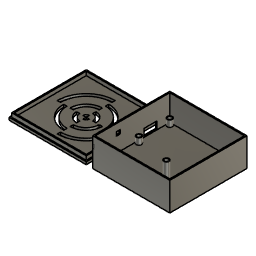
Fujitsu case new v2 (Autodesk Fusion 360 design; units mm, degrees)
Autodesk Fusion 360 part; units mm, degrees
note: some values were not read from the file. Set by a fixed rule: which sketch regions a step uses.
sketch "Sketch1" plane through (0, 0, 0) normal (0, 0, 1) x (1, 0, 0)
  line L0 (30, -30) -> (-30, -30)
  line L1 (-30, -30) -> (-30, 30)
  line L2 (-30, 30) -> (30, 30)
  line L3 (30, 30) -> (30, -30)
  line L4 (30, -30) -> (-30, 30) construction
  line L5 (-30, -30) -> (30, 30) construction
  dimension "d1" = 60
  dimension "d2" = 60
  constraint horizontal L0
  constraint perpendicular L0 L1
  constraint parallel L0 L2
  constraint parallel L1 L3
  constraint coincident L4 origin
  constraint coincident L5 origin
  measures "d1" distance of L1.end L2.end
  measures "d2" distance of L0.end L1.end
extrude "Extrude1" add sketch "Sketch1" along normal blind 2 makes body 1
sketch "Sketch2" plane through (0, 0, 2) normal (0, 0, 1) x (-1, 0, 0)
  line L0 (-30, -30) -> (30, -30)
  line L1 (30, -30) -> (30, 30)
  line L2 (30, 30) -> (-30, 30)
  line L3 (-30, 30) -> (-30, -30)
  line L4 (30, -30) -> (-30, -30)
  line L5 (-30, -30) -> (-30, 30)
  line L6 (-30, 30) -> (30, 30)
  line L7 (30, 30) -> (30, -30)
  line L8 (29, -29) -> (-29, -29)
  line L9 (-29, -29) -> (-29, 29)
  line L10 (-29, 29) -> (29, 29)
  line L11 (29, 29) -> (29, -29)
  constraint horizontal L4
  constraint vertical L5
  constraint horizontal L6
  constraint vertical L7
  constraint coincident L2.end L3.start
  constraint coincident L0.end L1.start
  constraint horizontal L8
  constraint vertical L9
  constraint horizontal L10
  constraint vertical L11
extrude "Extrude2" add sketch "Sketch2" along normal blind 20 bodies 1
sketch "Sketch3" plane through (0, 0, 2) normal (0, 0, 1) x (-1, 0, 0)
  line L0 (-29, 29) -> (-29, -29)
  line L1 (-29, -29) -> (29, -29)
  line L2 (29, -29) -> (29, 29)
  line L3 (29, 29) -> (-29, 29)
  circle A0 centre (27, -27) radius 2
  circle A1 centre (27, -27) radius 1.5
  line L4 (27, -27) -> (27, -3)
  circle A2 centre (27, -3) radius 1.5
  circle A3 centre (27, -3) radius 2
  line L5 (27, -27) -> (-19, -27)
  circle A4 centre (-19, -27) radius 1.5
  circle A5 centre (-19, -27) radius 2
  line L6 (27, -3) -> (-19, -3)
  circle A6 centre (-19, -3) radius 1.5
  circle A7 centre (-19, -3) radius 2
  dimension "d7" = 4
  dimension "d8" = 3
  dimension "d9" = 24
  dimension "d10" = 3
  dimension "d11" = 4
  dimension "d12" = 46
  dimension "d13" = 3
  dimension "d14" = 4
  dimension "d15" = 46
  dimension "d16" = 3
  dimension "d17" = 4
  constraint concentric A0 A1
  constraint coincident A0.centre A1.centre
  constraint parallel L2 L4
  constraint coincident L4.end A2.centre
  constraint concentric A2 A3
  constraint perpendicular L4 L5
  constraint coincident L5.end A4.centre
  constraint concentric A4 A5
  constraint perpendicular L4 L6
  constraint coincident L6.end A6.centre
  constraint concentric A6 A7
  measures "d7" diameter of A0
  measures "d8" diameter of A1
  measures "d9" distance of A0.centre L4.end
  measures "d10" diameter of A2
  measures "d11" diameter of A3
  measures "d12" distance of A0.centre L5.end
  measures "d13" diameter of A4
  measures "d14" diameter of A5
  measures "d15" distance of L4.end L6.end
  measures "d16" diameter of A6
  measures "d17" diameter of A7
extrude "Extrude3" add sketch "Sketch3" along normal blind 5 separate body contours A5 | L4 A2 A3 L6 | A0 A1 L4 L5 | L4 A2 A3 L6 | A0 A1 L4 L5 | A7 makes body 2 at (-28.9901, 3.1991, 3.6667) makes body 3 at (-28.9901, 27.1991, 3.6667) makes body 4 at (17.0025, 3.0997, 5.3333) makes body 5 at (17.0099, 27.1991, 3.6667)
sketch "Sketch4" plane through (-30, 0, 0) normal (-1, 0, 0) x (0, -1, 0)
  line L0 (-30, 0) -> (30, 0)
  line L1 (30, 0) -> (30, 22)
  line L2 (30, 22) -> (-30, 22)
  line L3 (-30, 22) -> (-30, 0)
  line L4 (-30, 0) -> (-14, 0)
  line L5 (-14, 0) -> (-14, 7)
  line L6 (-14, 7) -> (-14, 7.5)
  line L7 (-14, 7.5) -> (-19, 7.5)
  line L8 (-19, 7.5) -> (-9, 7.5)
  line L9 (-9, 7.5) -> (-9, 2.5)
  line L10 (-9, 2.5) -> (-19, 2.5)
  line L11 (-19, 2.5) -> (-19, 7.5)
  dimension "d20" = 16
  dimension "d21" = 7
  dimension "d22" = 0.5
  dimension "d23" = 5
  dimension "d24" = 10
  dimension "d25" = 5
  constraint coincident L0.start L3.end
  constraint perpendicular L3 L4
  constraint perpendicular L4 L5
  constraint parallel L5 L6
  constraint perpendicular L6 L7
  constraint horizontal L8
  constraint vertical L9
  constraint horizontal L10
  constraint vertical L11
  measures "d20" distance of L0.start L4.end
  measures "d21" distance of L4.end L5.end
  measures "d22" distance of L5.end L6.end
  measures "d23" distance of L6.end L7.end
  measures "d24" distance of L7.end L8.end
  measures "d25" distance of L7.end L10.end
extrude "Extrude4" cut sketch "Sketch4" against normal blind 1 contours L5 L6 L7 L8 L10 L11 | L5 L6 L8 L9 L10 bodies 1
extrude "Extrude5" cut 1 faces at (-29.6667, 15.6667, 7.5) along direction (0, 0, 1) blind 0.5 on bodies 1 bodies 1
sketch "Sketch5" plane through (0, 0, 2) normal (0, 0, 1) x (-1, 0, 0)
  line L0 (-29, 29) -> (-29, -29)
  line L1 (-29, -29) -> (29, -29)
  line L2 (29, -29) -> (29, 29)
  line L3 (29, 29) -> (-29, 29)
  line L4 (22, 29) -> (29, 29)
  line L5 (22, 29) -> (22, 27)
  circle A0 centre (22, 27) radius 2
  circle A1 centre (22, 27) radius 1.5
  line L6 (29, 29) -> (29, 11)
  line L7 (29, 11) -> (-7.9977, 10.5843)
  circle A2 centre (-7.9977, 10.5843) radius 1.5
  circle A3 centre (-7.9977, 10.5843) radius 2
  dimension "d31" = 7
  dimension "d32" = 2
  dimension "d33" = 4
  dimension "d34" = 3
  dimension "d35" = 18
  dimension "d37" = 37
  dimension "d38" = 3
  dimension "d39" = 4
  constraint coincident L2.end L3.start
  constraint perpendicular L2 L4
  constraint perpendicular L4 L5
  constraint coincident L5.end A0.centre
  constraint concentric A0 A1
  constraint perpendicular L4 L6
  constraint coincident L7.end A2.centre
  constraint concentric A2 A3
  measures "d31" distance of L4.start L2.end
  measures "d32" distance of L4.start L5.end
  measures "d33" diameter of A0
  measures "d34" diameter of A1
  measures "d35" distance of L2.end L6.end
  measures "d37" distance of L6.end L7.end
  measures "d38" diameter of A2
  measures "d39" diameter of A3
extrude "Extrude6" add sketch "Sketch5" along normal blind 13 separate body contours A0 | A3 makes body 6 at (-23.9975, -26.9003, 6.3333) makes body 7 at (6.0076, -10.7834, 10.6667)
sketch "Sketch6" plane through (0, 0, 2) normal (0, 0, 1) x (-1, 0, 0)
  line L0 (-29, 29) -> (-29, -29)
  line L1 (-29, -29) -> (29, -29)
  line L2 (29, -29) -> (29, 29)
  line L3 (29, 29) -> (-29, 29)
  line L4 (29, 29) -> (2, 29)
  line L5 (2, 29) -> (2, 26)
  circle A0 centre (2, 26) radius 1.5
  dimension "d42" = 27
  dimension "d43" = 3
  dimension "d44" = 3
  constraint coincident L2.end L3.start
  constraint perpendicular L2 L4
  constraint perpendicular L3 L5
  constraint coincident L5.end A0.centre
  measures "d42" distance of L2.end L4.end
  measures "d43" distance of L4.end L5.end
  measures "d44" diameter of A0
extrude "Extrude7" cut sketch "Sketch6" against normal blind 5 contours A0 bodies 1
sketch "Sketch7" plane through (-30, 0, 0) normal (-1, 0, 0) x (0, -1, 0)
  line L0 (-9, 8) -> (-9, 2.5)
  line L1 (-9, 2.5) -> (-19, 2.5)
  line L2 (-19, 2.5) -> (-19, 8)
  line L3 (-19, 8) -> (-9, 8)
  line L4 (-30, 0) -> (30, 0)
  line L5 (30, 0) -> (30, 22)
  line L6 (30, 22) -> (-30, 22)
  line L7 (-30, 22) -> (-30, 0)
  line L8 (30, 0) -> (28, 0)
  line L9 (28, 0) -> (28, 15)
  line L10 (29.5, 13.5) -> (26.5, 13.5)
  line L11 (26.5, 13.5) -> (26.5, 16.5)
  line L12 (26.5, 16.5) -> (29.5, 16.5)
  line L13 (29.5, 16.5) -> (29.5, 13.5)
  line L14 (29.5, 13.5) -> (26.5, 16.5) construction
  line L15 (26.5, 13.5) -> (29.5, 16.5) construction
  line L16 (29.5, 15) -> (9.5, 15)
  line L17 (9.5, 15) -> (11, 15)
  line L18 (12.5, 13.5) -> (9.5, 13.5)
  line L19 (9.5, 13.5) -> (9.5, 16.5)
  line L20 (9.5, 16.5) -> (12.5, 16.5)
  line L21 (12.5, 16.5) -> (12.5, 13.5)
  line L22 (12.5, 13.5) -> (9.5, 16.5) construction
  line L23 (9.5, 13.5) -> (12.5, 16.5) construction
  point P0 (28, 15)
  point P1 (11, 15)
  dimension "d47" = 15
  dimension "d48" = 3
  dimension "d49" = 3
  dimension "d50" = 20
  dimension "d51" = 1.5
  dimension "d52" = 3
  dimension "d53" = 3
  constraint coincident L4.end L5.start
  constraint coincident L4 L8.end
  constraint perpendicular L5 L8
  constraint perpendicular L6 L9
  constraint horizontal L10
  constraint perpendicular L10 L11
  constraint parallel L10 L12
  constraint parallel L11 L13
  constraint coincident L14 P0
  constraint coincident L15 P0
  constraint coincident P0 L9.end
  constraint midpoint L13 L16.start
  constraint perpendicular L13 L16
  constraint parallel L16 L17
  constraint horizontal L18
  constraint perpendicular L18 L19
  constraint parallel L18 L20
  constraint parallel L19 L21
  constraint coincident L22 P1
  constraint coincident L23 P1
  constraint coincident P1 L17.end
  measures "d47" distance of L8.end P0
  measures "d48" distance of L11.end L12.end
  measures "d49" distance of L10.end L11.end
  measures "d50" distance of L16.start L16.end
  measures "d51" distance of L16.end P1
  measures "d52" distance of L19.end L20.end
  measures "d53" distance of L18.end L19.end
extrude "Extrude8" cut sketch "Sketch7" against normal blind 1 contours L9 L10 L11 L16 | L9 L10 L13 L16 | L11 L12 L13 L16 | L16 L17 L18 L19 L21 | L16 L17 L19 L20 L21 bodies 1
sketch "Sketch8" plane through (0, 0, 0) normal (0, 0, 1) x (1, 0, 0)
  line L0 (-35, -30) -> (-95, -30)
  line L1 (-95, -30) -> (-95, 30)
  line L2 (-95, 30) -> (-35, 30)
  line L3 (-35, 30) -> (-35, -30)
  dimension "d56" = 60
  constraint horizontal L0
  constraint vertical L1
  constraint horizontal L2
  constraint vertical L3
  measures "d56" distance of L0.start L0.end
extrude "Extrude9" add sketch "Sketch8" along normal blind 2 separate body makes body 8
sketch "Sketch9" plane through (0, 0, 2) normal (0, 0, 1) x (-1, 0, 0)
  line L0 (35, -30) -> (95, -30)
  line L1 (95, -30) -> (95, 30)
  line L2 (95, 30) -> (35, 30)
  line L3 (35, 30) -> (35, -30)
  line L4 (35, 30) -> (36, 30)
  line L5 (36, 29) -> (94, 29)
  line L6 (94, 29) -> (94, -29)
  line L7 (94, -29) -> (36, -29)
  line L8 (36, -29) -> (36, 29)
  line L9 (37, 28) -> (93, 28)
  line L10 (93, 28) -> (93, -28)
  line L11 (93, -28) -> (37, -28)
  line L12 (37, -28) -> (37, 28)
  dimension "d59" = 1
  constraint coincident L2.end L3.start
  constraint perpendicular L3 L4
  constraint horizontal L5
  constraint vertical L6
  constraint horizontal L7
  constraint vertical L8
  constraint horizontal L9
  constraint vertical L10
  constraint horizontal L11
  constraint vertical L12
  measures "d59" distance of L2.end L4.end
extrude "Extrude10" add sketch "Sketch9" along normal blind 3 contours L5 L6 L7 L8 bodies 8
sketch "Sketch10" plane through (0, 0, 2) normal (0, 0, 1) x (-1, 0, 0)
  line L0 (93, -28) -> (93, 28)
  line L1 (93, 28) -> (37, 28)
  line L2 (37, 28) -> (37, -28)
  line L3 (37, -28) -> (93, -28)
  circle A0 centre (65, 0) radius 2.5
  circle A1 centre (65, 0) radius 5
  circle A2 centre (65, 0) radius 7.5
  circle A3 centre (65, 0) radius 10
  circle A4 centre (65, 0) radius 25
  circle A5 centre (65, 0) radius 12.5
  circle A6 centre (65, 0) radius 15
  circle A7 centre (65, 0) radius 17.5
  circle A8 centre (65, 0) radius 20
  circle A9 centre (65, 0) radius 7.5
  circle A10 centre (65, 0) radius 22.5
  line L4 (65, 0) -> (65, -25)
  line L5 (65, 0) -> (90, 0)
  line L6 (65, 0) -> (65, 25)
  line L7 (65, 0) -> (40, 0)
  dimension "d62" = 5
  dimension "d63" = 10
  dimension "d64" = 15
  dimension "d65" = 20
  dimension "d66" = 50
  dimension "d67" = 25
  dimension "d68" = 30
  dimension "d69" = 35
  dimension "d70" = 40
  dimension "d71" = 15
  dimension "d72" = 45
  constraint concentric A0 A1
  constraint concentric A1 A2
  constraint concentric A1 A3
  constraint concentric A2 A4
  constraint concentric A2 A5
  constraint concentric A2 A6
  constraint concentric A2 A7
  constraint concentric A3 A8
  constraint concentric A0 A9
  constraint concentric A2 A10
  constraint coincident A0.centre A1.centre
  constraint coincident A4 L4.end
  constraint vertical L4
  constraint coincident A4 L5.end
  constraint perpendicular L4 L5
  constraint coincident A4 L6.end
  constraint perpendicular L5 L6
  constraint coincident A4 L7.end
  constraint perpendicular L6 L7
  measures "d62" diameter of A0
  measures "d63" diameter of A1
  measures "d64" diameter of A2
  measures "d65" diameter of A3
  measures "d66" diameter of A4
  measures "d67" diameter of A5
  measures "d68" diameter of A6
  measures "d69" diameter of A7
  measures "d70" diameter of A8
  measures "d71" diameter of A9
  measures "d72" diameter of A10
extrude "Extrude11" cut sketch "Sketch10" against normal blind 3 contours A0 L4 L5 | A0 L6 L7 | A1 A2 A9 L5 L6 | A1 A2 A9 L4 L7 | A3 A5 L4 L5 | A3 A5 L6 L7 | A6 A7 L5 L6 | A6 A7 L4 L7 | A8 A10 L4 L5 | A8 A10 L6 L7 bodies 8
